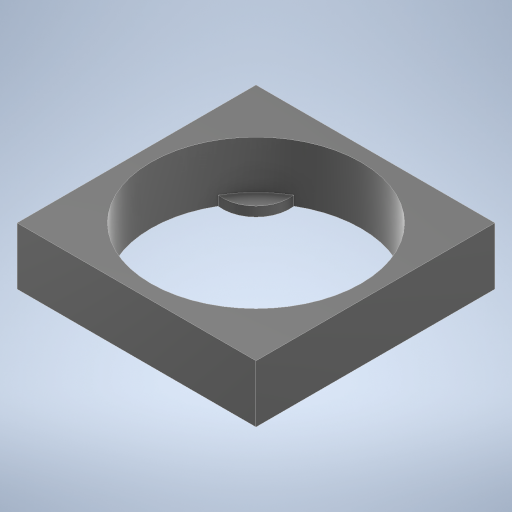
# Autodesk Inventor part: spacers_base
Saved by Autodesk Inventor 2024.2 (Build 282272000, 272)
## iProperties
Created: 2023-10-06
Part Number: spacers_base
Material: Generic
Document SubType Name: Modeling
Designer: gwi5013
Density: 1 g/cm^3
Appearance: Smooth - Black
Author: gwi5013
Autodesk Inventor part; units mm, degrees
ref_plane "YZ Plane" through (0, 0, 0) normal (1, 0, 0) x (0, 1, 0)
ref_plane "XZ Plane" through (0, 0, 0) normal (0, 1, 0) x (-1, 0, 0)
ref_plane "XY Plane" through (0, 0, 0) normal (0, 0, 1) x (1, 0, 0)
sketch "Sketch1" plane through (0, 0, 0) normal (0, 1, 0) x (-1, 0, 0)
  line L0 (0, 0) -> (25, 0)
  line L1 (25, 0) -> (25, -25)
  line L2 (25, -25) -> (0, -25)
  line L3 (0, -25) -> (0, 0)
  circle A0 centre (12.5, -12.5) radius 11
  circle A1 centre (3.5, -3.5) radius 3.5
  circle A2 centre (3.5, -21.5) radius 3.5
  circle A3 centre (21.5, -21.5) radius 3.5
  circle A4 centre (21.5, -3.5) radius 3.5
  line L4 (25, -12.5) -> (0, -12.5) construction
  line L5 (12.5, -25) -> (12.5, 0) construction
  point P0 (6.9634, -2.995)
  point P1 (2.995, -6.9634)
  point P2 (18.0366, -2.995)
  point P3 (22.005, -6.9634)
  point P4 (6.9634, -22.005)
  point P5 (2.995, -18.0366)
  point P6 (22.005, -18.0366)
  point P7 (18.0366, -22.005)
  point P8 (0, -3.5)
  point P9 (3.5, 0)
  point P10 (25, -3.5)
  point P11 (21.5, 0)
  point P12 (0, -21.5)
  point P13 (3.5, -25)
  point P14 (21.5, -25)
  point P15 (25, -21.5)
  dimension "cellRadius" = 22
  dimension "catcherRadius" = 7
  dimension "d27" = 7
  dimension "d28" = 7
  dimension "d29" = 7
  dimension "d36" = 25
  dimension "d37" = 25
  constraints: 12 end point, 8 tangent, 5 centre point, 4 midpoint, 2 line through centre, 2 parallel, 1 horizontal, 1 perpendicular
  measures "cellRadius" diameter of A0
  measures "catcherRadius" diameter of A1
  measures "d27" diameter of A2
  measures "d28" diameter of A3
  measures "d29" diameter of A4
  measures "d36" distance of L2.end L0.start
  measures "d37" distance of L0.start L0.end
extrude "thickness" add sketch "Sketch1" along normal blind 6 contours L0 A1 L3 | L0 A4 A0 A1 | A1 A0 | A1 A0 A2 L3 | L0 L1 A4 | A4 A0 | A2 L2 L3 | A2 A0 | L1 A3 A0 A4 | A2 A0 A3 L2 | A3 A0 | L1 L2 A3 picked at (3.6063, -3.4216) picked at (21.3937, -3.4216) picked at (3.4216, -21.3937) picked at (21.3937, -21.5784)
extrude "catcher" add sketch "Sketch1" along normal blind 1 contours L0 A1 L3 | A1 A0 | L0 L1 A4 | A4 A0 | A1 A0 | A2 L2 L3 | A2 A0 | A0 A4 | A2 A0 | A3 A0 | L1 L2 A3 | A0 A3
equation "\"d27\" = catcherRadius"
equation "\"d28\" = catcherRadius"
equation "\"d29\" = catcherRadius"
equation "\"d36\" = width"
equation "\"d37\" = width"
equation "\"catcherHeight\" = 0.166667 * spacerHeight"
equation "\"width\" = 25"
equation "\"spacerHeight\" = 6"
body "Solid2"
